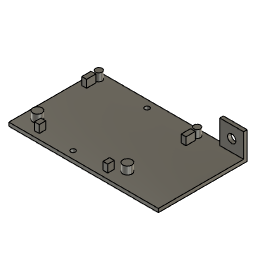
rasp (Autodesk Fusion 360 design; units mm, degrees)
Autodesk Fusion 360 part; units mm, degrees
sketch "Sketch1" plane through (0, 0, 0) normal (0, 0, 1) x (1, 0, 0)
  line L0 (-47.74, 37.25) -> (47.74, 37.25)
  line L1 (47.74, 37.25) -> (47.74, -37.25)
  line L2 (47.74, -37.25) -> (-47.74, -37.25)
  line L3 (-47.74, -37.25) -> (-47.74, 37.25)
  line L4 (-47.74, 37.25) -> (47.74, -37.25) construction
  line L5 (47.74, 37.25) -> (-47.74, -37.25) construction
  circle A0 centre (41.24, 31.75) radius 2.78
  circle A1 centre (-41.24, 31.75) radius 2.78
  circle A2 centre (37.74, -23.25) radius 3.84
  circle A3 centre (-37.74, -23.25) radius 3.84
  line L6 (-30.74, -27.25) -> (-26.74, -27.25)
  line L7 (-26.74, -27.25) -> (-26.74, -33.25)
  line L8 (-26.74, -33.25) -> (-30.74, -33.25)
  line L9 (-30.74, -33.25) -> (-30.74, -27.25)
  line L10 (26.74, -27.25) -> (30.74, -27.25)
  line L11 (30.74, -27.25) -> (30.74, -33.25)
  line L12 (30.74, -33.25) -> (26.74, -33.25)
  line L13 (26.74, -33.25) -> (26.74, -27.25)
  line L14 (39.74, 27.75) -> (43.74, 27.75)
  line L15 (43.74, 27.75) -> (43.74, 19.95)
  line L16 (43.74, 19.95) -> (39.74, 19.95)
  line L17 (39.74, 19.95) -> (39.74, 27.75)
  line L18 (-43.74, 27.75) -> (-39.74, 27.75)
  line L19 (-39.74, 27.75) -> (-39.74, 19.95)
  line L20 (-39.74, 19.95) -> (-43.74, 19.95)
  line L21 (-43.74, 19.95) -> (-43.74, 27.75)
  point P0 (40, 20)
  dimension "d2" = 95.48
  dimension "d3" = 74.5
  dimension "d4" = 5.56
  dimension "d5" = 5.56
  dimension "d6" = 7.68
  dimension "d7" = 7.68
  dimension "d8" = 5.5
  dimension "d9" = 6.5
  dimension "d10" = 6.5
  dimension "d11" = 5.5
  dimension "d12" = 14
  dimension "d13" = 10
  dimension "d14" = 10
  dimension "d15" = 14
  dimension "d22" = 4
  dimension "d23" = 6
  dimension "d24" = 4
  dimension "d25" = 7
  dimension "d26" = 4
  dimension "d27" = 6
  dimension "d28" = 7
  dimension "d29" = 4
  dimension "d30" = 4
  dimension "d31" = 7.8
  dimension "d32" = 4
  dimension "d33" = 4
  dimension "d34" = 4
  dimension "d35" = 7.8
  dimension "d36" = 4
  dimension "d37" = 4
  constraint horizontal L0
  constraint perpendicular L0 L1
  constraint parallel L0 L2
  constraint parallel L1 L3
  constraint coincident L4 origin
  constraint coincident L5 origin
  constraint horizontal L6
  constraint vertical L7
  constraint horizontal L8
  constraint vertical L9
  constraint horizontal L10
  constraint vertical L11
  constraint horizontal L12
  constraint vertical L13
  constraint horizontal L14
  constraint vertical L15
  constraint horizontal L16
  constraint vertical L17
  constraint horizontal L18
  constraint vertical L19
  constraint horizontal L20
  constraint vertical L21
  measures "d2" distance of L1.end L2.end
  measures "d3" distance of L0.end L1.end
  measures "d4" diameter of A0
  measures "d5" diameter of A1
  measures "d6" diameter of A2
  measures "d7" diameter of A3
  measures "d8" distance of L0 A1.centre
  measures "d9" distance of L3 A1.centre
  measures "d10" distance of L1 A0.centre
  measures "d11" distance of L0 A0.centre
  measures "d12" distance of L2 A2.centre
  measures "d13" distance of L1 A2.centre
  measures "d14" distance of L3 A3.centre
  measures "d15" distance of L2 A3.centre
  measures "d22" distance of L6.start L6.end
  measures "d23" distance of L6.start L8.end
  measures "d24" distance of L2 L8
  measures "d25" distance of A3.centre L9
  measures "d26" distance of L10.start L10.end
  measures "d27" distance of L10.start L12.end
  measures "d28" distance of A2.centre L11
  measures "d29" distance of L2 L12
  measures "d30" distance of L14.start L14.end
  measures "d31" distance of L14.start L16.end
  measures "d32" distance of L1 L15
  measures "d33" distance of A0.centre L14
  measures "d34" distance of L18.start L18.end
  measures "d35" distance of L18.start L20.end
  measures "d36" distance of L3 L21
  measures "d37" distance of A1.centre L18
extrude "Extrude1" add sketch "Sketch1" along normal blind 9.5 contours A0 | A1 | A2 | A3 | L6 L7 L8 L9 | L10 L11 L12 L13 | L14 L15 L16 L17 | L18 L19 L20 L21 makes body 1 at (41.5609, -23.6323, 6.3333) makes body 2 at (-33.9191, -23.6323, 6.3333) makes body 3 at (30.74, -29.25, 3.1667) makes body 4 at (-26.74, -29.25, 3.1667) makes body 5 at (44.0062, 31.4732, 6.3333) makes body 6 at (-38.4738, 31.4732, 6.3333) makes body 7 at (43.74, 25.15, 3.1667) makes body 8 at (-39.74, 25.15, 6.3333)
extrude "Extrude2" add sketch "Sketch1" along normal blind 3 bodies 1 2 3 4 5 6 7 8
sketch "Sketch6" plane through (0, 0, 3) normal (0, 0, 1) x (-1, 0, 0)
  circle A0 centre (41.24, -31.75) radius 2.78
  circle A1 centre (37.74, 23.25) radius 3.84
  line L0 (26.74, 33.25) -> (30.74, 33.25)
  line L1 (30.74, 33.25) -> (30.74, 27.25)
  line L2 (30.74, 27.25) -> (26.74, 27.25)
  line L3 (26.74, 27.25) -> (26.74, 33.25)
  circle A2 centre (-37.74, 23.25) radius 3.84
  line L4 (-30.74, 33.25) -> (-26.74, 33.25)
  line L5 (-26.74, 33.25) -> (-26.74, 27.25)
  line L6 (-26.74, 27.25) -> (-30.74, 27.25)
  line L7 (-30.74, 27.25) -> (-30.74, 33.25)
  line L8 (-43.74, -19.95) -> (-39.74, -19.95)
  line L9 (-39.74, -19.95) -> (-39.74, -27.75)
  line L10 (-39.74, -27.75) -> (-43.74, -27.75)
  line L11 (-43.74, -27.75) -> (-43.74, -19.95)
  circle A3 centre (-41.24, -31.75) radius 2.78
  line L12 (39.74, -19.95) -> (43.74, -19.95)
  line L13 (43.74, -19.95) -> (43.74, -27.75)
  line L14 (43.74, -27.75) -> (39.74, -27.75)
  line L15 (39.74, -27.75) -> (39.74, -19.95)
  line L16 (47.74, 37.25) -> (-47.74, 37.25)
  line L17 (-47.74, 37.25) -> (-47.74, -37.25)
  line L18 (-47.74, -37.25) -> (47.74, -37.25)
  line L19 (47.74, -37.25) -> (47.74, 37.25)
  line L20 (-145.7882, -27) -> (145.7882, -27)
  line L21 (145.7882, -27) -> (145.7882, 27)
  line L22 (145.7882, 27) -> (-145.7882, 27)
  line L23 (-145.7882, 27) -> (-145.7882, -27)
  line L24 (-145.7882, -27) -> (145.7882, 27) construction
  line L25 (145.7882, -27) -> (-145.7882, 27) construction
  circle A4 centre (0, -31) radius 2
  line L26 (-20, 0) -> (-2.5, 0)
  circle A5 centre (0, 31) radius 2
  point P0 (0, -31)
  dimension "d42" = 54
  dimension "d44" = 4
  dimension "d47" = 4
  dimension "d50" = 31
  constraint horizontal L20
  constraint perpendicular L20 L21
  constraint parallel L20 L22
  constraint parallel L21 L23
  constraint coincident L24 origin
  constraint coincident L25 origin
  constraint vertical origin A4.centre
  constraint coincident P0 A4.centre
  constraint symmetric A4 L26 A5
  measures "d42" distance of L20.start L22.end
  measures "d44" distance of L20 P0
  measures "d47" diameter of A4
  measures "d50" distance of origin A4.centre
move_face "OffsetFaces1" offset -0.5 2 faces at (-28.0733, -33.25, 5.1667) (29.4067, -33.25, 5.1667) on bodies 1
extrude "Extrude3" cut sketch "Sketch6" against normal blind 5 contours A4 | A5 bodies 1
extrude "Extrude5" add 1 faces at (47.74, 12.4167, 1) along direction (1, 0, 0) blind 30 on bodies 1 bodies 1
sketch "Sketch11" plane through (0, 37.25, 0) normal (0, 1, 0) x (-1, 0, 0)
  line L0 (-77.74, 0) -> (47.74, 0)
  line L1 (47.74, 0) -> (47.74, 3)
  line L2 (47.74, 3) -> (-77.74, 3)
  line L3 (-77.74, 3) -> (-77.74, 0)
  line L4 (-77.74, 3) -> (-57.74, 3)
  line L5 (-57.74, 3) -> (-57.74, 23)
  line L6 (-57.74, 23) -> (-77.74, 23)
  line L7 (-77.74, 23) -> (-77.74, 3)
  circle A0 centre (-67.74, 13) radius 3.5
  dimension "d56" = 20
  dimension "d57" = 20
  dimension "d58" = 7
  dimension "d59" = 10
  dimension "d60" = 10
  constraint horizontal L4
  constraint vertical L5
  constraint horizontal L6
  constraint vertical L7
  constraint coincident L2.end L3.start
  measures "d56" distance of L2.end L6.end
  measures "d57" distance of L5.end L6.end
  measures "d58" diameter of A0
  measures "d59" distance of L5 A0.centre
  measures "d60" distance of L6 A0.centre
extrude "Extrude6" add sketch "Sketch11" against normal blind 3 contours L2 L4 L5 L6 L7 bodies 1
